Autodesk Inventor part; units mm, degrees
(part 2 of 2)
sketch "ShorterHoneycomb" plane through (90.804, 0, 48.8878) normal (1, 0, 0) x (0, 0, -1)
  line L0 (0, 131) -> (113, 131)
  line L1 (113, 131) -> (113, 0)
  line L2 (113, 0) -> (0, 0)
  line L3 (0, 0) -> (0, 131)
  line L4 (4, 131) -> (109, 131)
  line L5 (109, 131) -> (109, 0)
  line L6 (109, 0) -> (4, 0)
  line L7 (4, 0) -> (4, 131)
  line L8 (15.2583, 115) -> (7.7528, 115)
  line L9 (7.7528, 115) -> (4, 121.5)
  line L10 (4, 121.5) -> (7.7528, 128)
  line L11 (7.7528, 128) -> (15.2583, 128)
  line L12 (15.2583, 128) -> (19.0111, 121.5)
  line L13 (19.0111, 121.5) -> (15.2583, 115)
  line L14 (27.094, 107.5) -> (19.5885, 107.5)
  line L15 (19.5885, 107.5) -> (15.8357, 114)
  line L16 (15.8357, 114) -> (19.5885, 120.5)
  line L17 (19.5885, 120.5) -> (27.094, 120.5)
  line L18 (27.094, 120.5) -> (30.8468, 114)
  line L19 (30.8468, 114) -> (27.094, 107.5)
  line L20 (0, 131) -> (113, 131) projected
  line L21 (19.0111, 121.5) -> (19.5885, 120.5) construction
  line L22 (15.2583, 115) -> (15.8357, 114) construction
  line L23 (15.2583, 100) -> (7.7528, 100)
  line L24 (7.7528, 100) -> (4, 106.5)
  line L25 (4, 106.5) -> (7.7528, 113)
  line L26 (7.7528, 113) -> (15.2583, 113)
  line L27 (15.2583, 113) -> (19.0111, 106.5)
  line L28 (19.0111, 106.5) -> (15.2583, 100)
  line L29 (27.094, 92.5) -> (19.5885, 92.5)
  line L30 (19.5885, 92.5) -> (15.8357, 99)
  line L31 (15.8357, 99) -> (19.5885, 105.5)
  line L32 (19.5885, 105.5) -> (27.094, 105.5)
  line L33 (27.094, 105.5) -> (30.8468, 99)
  line L34 (30.8468, 99) -> (27.094, 92.5)
  line L35 (19.0111, 106.5) -> (19.5885, 105.5) construction
  line L36 (15.2583, 100) -> (15.8357, 99) construction
  line L37 (15.2583, 85) -> (7.7528, 85)
  line L38 (7.7528, 85) -> (4, 91.5)
  line L39 (4, 91.5) -> (7.7528, 98)
  line L40 (7.7528, 98) -> (15.2583, 98)
  line L41 (15.2583, 98) -> (19.0111, 91.5)
  line L42 (19.0111, 91.5) -> (15.2583, 85)
  line L43 (27.094, 77.5) -> (19.5885, 77.5)
  line L44 (19.5885, 77.5) -> (15.8357, 84)
  line L45 (15.8357, 84) -> (19.5885, 90.5)
  line L46 (19.5885, 90.5) -> (27.094, 90.5)
  line L47 (27.094, 90.5) -> (30.8468, 84)
  line L48 (30.8468, 84) -> (27.094, 77.5)
  line L49 (19.0111, 91.5) -> (19.5885, 90.5) construction
  line L50 (15.2583, 85) -> (15.8357, 84) construction
  line L51 (15.2583, 70) -> (7.7528, 70)
  line L52 (7.7528, 70) -> (4, 76.5)
  line L53 (4, 76.5) -> (7.7528, 83)
  line L54 (7.7528, 83) -> (15.2583, 83)
  line L55 (15.2583, 83) -> (19.0111, 76.5)
  line L56 (19.0111, 76.5) -> (15.2583, 70)
  line L57 (27.094, 62.5) -> (19.5885, 62.5)
  line L58 (19.5885, 62.5) -> (15.8357, 69)
  line L59 (15.8357, 69) -> (19.5885, 75.5)
  line L60 (19.5885, 75.5) -> (27.094, 75.5)
  line L61 (27.094, 75.5) -> (30.8468, 69)
  line L62 (30.8468, 69) -> (27.094, 62.5)
  line L63 (19.0111, 76.5) -> (19.5885, 75.5) construction
  line L64 (15.2583, 70) -> (15.8357, 69) construction
  line L65 (15.2583, 55) -> (7.7528, 55)
  line L66 (7.7528, 55) -> (4, 61.5)
  line L67 (4, 61.5) -> (7.7528, 68)
  line L68 (7.7528, 68) -> (15.2583, 68)
  line L69 (15.2583, 68) -> (19.0111, 61.5)
  line L70 (19.0111, 61.5) -> (15.2583, 55)
  line L71 (27.094, 47.5) -> (19.5885, 47.5)
  line L72 (19.5885, 47.5) -> (15.8357, 54)
  line L73 (15.8357, 54) -> (19.5885, 60.5)
  line L74 (19.5885, 60.5) -> (27.094, 60.5)
  line L75 (27.094, 60.5) -> (30.8468, 54)
  line L76 (30.8468, 54) -> (27.094, 47.5)
  line L77 (19.0111, 61.5) -> (19.5885, 60.5) construction
  line L78 (15.2583, 55) -> (15.8357, 54) construction
  line L79 (15.2583, 40) -> (7.7528, 40)
  line L80 (7.7528, 40) -> (4, 46.5)
  line L81 (4, 46.5) -> (7.7528, 53)
  line L82 (7.7528, 53) -> (15.2583, 53)
  line L83 (15.2583, 53) -> (19.0111, 46.5)
  line L84 (19.0111, 46.5) -> (15.2583, 40)
  line L85 (27.094, 32.5) -> (19.5885, 32.5)
  line L86 (19.5885, 32.5) -> (15.8357, 39)
  line L87 (15.8357, 39) -> (19.5885, 45.5)
  line L88 (19.5885, 45.5) -> (27.094, 45.5)
  line L89 (27.094, 45.5) -> (30.8468, 39)
  line L90 (30.8468, 39) -> (27.094, 32.5)
  line L91 (19.0111, 46.5) -> (19.5885, 45.5) construction
  line L92 (15.2583, 40) -> (15.8357, 39) construction
  line L93 (15.2583, 25) -> (7.7528, 25)
  line L94 (7.7528, 25) -> (4, 31.5)
  line L95 (4, 31.5) -> (7.7528, 38)
  line L96 (7.7528, 38) -> (15.2583, 38)
  line L97 (15.2583, 38) -> (19.0111, 31.5)
  line L98 (19.0111, 31.5) -> (15.2583, 25)
  line L99 (27.094, 17.5) -> (19.5885, 17.5)
  line L100 (19.5885, 17.5) -> (15.8357, 24)
  line L101 (15.8357, 24) -> (19.5885, 30.5)
  line L102 (19.5885, 30.5) -> (27.094, 30.5)
  line L103 (27.094, 30.5) -> (30.8468, 24)
  line L104 (30.8468, 24) -> (27.094, 17.5)
  line L105 (19.0111, 31.5) -> (19.5885, 30.5) construction
  line L106 (15.2583, 25) -> (15.8357, 24) construction
  line L107 (15.2583, 10) -> (7.7528, 10)
  line L108 (7.7528, 10) -> (4, 16.5)
  line L109 (4, 16.5) -> (7.7528, 23)
  line L110 (7.7528, 23) -> (15.2583, 23)
  line L111 (15.2583, 23) -> (19.0111, 16.5)
  line L112 (19.0111, 16.5) -> (15.2583, 10)
  line L113 (27.094, 2.5) -> (19.5885, 2.5)
  line L114 (19.5885, 2.5) -> (15.8357, 9)
  line L115 (15.8357, 9) -> (19.5885, 15.5)
  line L116 (19.5885, 15.5) -> (27.094, 15.5)
  line L117 (27.094, 15.5) -> (30.8468, 9)
  line L118 (30.8468, 9) -> (27.094, 2.5)
  line L119 (19.0111, 16.5) -> (19.5885, 15.5) construction
  line L120 (15.2583, 10) -> (15.8357, 9) construction
  line L121 (38.9333, 115) -> (31.4278, 115)
  line L122 (31.4278, 115) -> (27.675, 121.5)
  line L123 (27.675, 121.5) -> (31.4278, 128)
  line L124 (31.4278, 128) -> (38.9333, 128)
  line L125 (38.9333, 128) -> (42.6861, 121.5)
  line L126 (42.6861, 121.5) -> (38.9333, 115)
  line L127 (50.769, 107.5) -> (43.2635, 107.5)
  line L128 (43.2635, 107.5) -> (39.5107, 114)
  line L129 (39.5107, 114) -> (43.2635, 120.5)
  line L130 (43.2635, 120.5) -> (50.769, 120.5)
  line L131 (50.769, 120.5) -> (54.5218, 114)
  line L132 (54.5218, 114) -> (50.769, 107.5)
  line L133 (42.6861, 121.5) -> (43.2635, 120.5) construction
  line L134 (38.9333, 115) -> (39.5107, 114) construction
  line L135 (38.9333, 100) -> (31.4278, 100)
  line L136 (31.4278, 100) -> (27.675, 106.5)
  line L137 (27.675, 106.5) -> (31.4278, 113)
  line L138 (31.4278, 113) -> (38.9333, 113)
  line L139 (38.9333, 113) -> (42.6861, 106.5)
  line L140 (42.6861, 106.5) -> (38.9333, 100)
  line L141 (50.769, 92.5) -> (43.2635, 92.5)
  line L142 (43.2635, 92.5) -> (39.5107, 99)
  line L143 (39.5107, 99) -> (43.2635, 105.5)
  line L144 (43.2635, 105.5) -> (50.769, 105.5)
  line L145 (50.769, 105.5) -> (54.5218, 99)
  line L146 (54.5218, 99) -> (50.769, 92.5)
  line L147 (42.6861, 106.5) -> (43.2635, 105.5) construction
  line L148 (38.9333, 100) -> (39.5107, 99) construction
  line L149 (38.9333, 85) -> (31.4278, 85)
  line L150 (31.4278, 85) -> (27.675, 91.5)
  line L151 (27.675, 91.5) -> (31.4278, 98)
  line L152 (31.4278, 98) -> (38.9333, 98)
  line L153 (38.9333, 98) -> (42.6861, 91.5)
  line L154 (42.6861, 91.5) -> (38.9333, 85)
  line L155 (50.769, 77.5) -> (43.2635, 77.5)
  line L156 (43.2635, 77.5) -> (39.5107, 84)
  line L157 (39.5107, 84) -> (43.2635, 90.5)
  line L158 (43.2635, 90.5) -> (50.769, 90.5)
  line L159 (50.769, 90.5) -> (54.5218, 84)
  line L160 (54.5218, 84) -> (50.769, 77.5)
  line L161 (42.6861, 91.5) -> (43.2635, 90.5) construction
  line L162 (38.9333, 85) -> (39.5107, 84) construction
  line L163 (38.9333, 70) -> (31.4278, 70)
  line L164 (31.4278, 70) -> (27.675, 76.5)
  line L165 (27.675, 76.5) -> (31.4278, 83)
  line L166 (31.4278, 83) -> (38.9333, 83)
  line L167 (38.9333, 83) -> (42.6861, 76.5)
  line L168 (42.6861, 76.5) -> (38.9333, 70)
  line L169 (50.769, 62.5) -> (43.2635, 62.5)
  line L170 (43.2635, 62.5) -> (39.5107, 69)
  line L171 (39.5107, 69) -> (43.2635, 75.5)
  line L172 (43.2635, 75.5) -> (50.769, 75.5)
  line L173 (50.769, 75.5) -> (54.5218, 69)
  line L174 (54.5218, 69) -> (50.769, 62.5)
  line L175 (42.6861, 76.5) -> (43.2635, 75.5) construction
  line L176 (38.9333, 70) -> (39.5107, 69) construction
  line L177 (38.9333, 55) -> (31.4278, 55)
  line L178 (31.4278, 55) -> (27.675, 61.5)
  line L179 (27.675, 61.5) -> (31.4278, 68)
  line L180 (31.4278, 68) -> (38.9333, 68)
  line L181 (38.9333, 68) -> (42.6861, 61.5)
  line L182 (42.6861, 61.5) -> (38.9333, 55)
  line L183 (50.769, 47.5) -> (43.2635, 47.5)
  line L184 (43.2635, 47.5) -> (39.5107, 54)
  line L185 (39.5107, 54) -> (43.2635, 60.5)
  line L186 (43.2635, 60.5) -> (50.769, 60.5)
  line L187 (50.769, 60.5) -> (54.5218, 54)
  line L188 (54.5218, 54) -> (50.769, 47.5)
  line L189 (42.6861, 61.5) -> (43.2635, 60.5) construction
  line L190 (38.9333, 55) -> (39.5107, 54) construction
  line L191 (38.9333, 40) -> (31.4278, 40)
  line L192 (31.4278, 40) -> (27.675, 46.5)
  line L193 (27.675, 46.5) -> (31.4278, 53)
  line L194 (31.4278, 53) -> (38.9333, 53)
  line L195 (38.9333, 53) -> (42.6861, 46.5)
  line L196 (42.6861, 46.5) -> (38.9333, 40)
  line L197 (50.769, 32.5) -> (43.2635, 32.5)
  line L198 (43.2635, 32.5) -> (39.5107, 39)
  line L199 (39.5107, 39) -> (43.2635, 45.5)
  line L200 (43.2635, 45.5) -> (50.769, 45.5)
  line L201 (50.769, 45.5) -> (54.5218, 39)
  line L202 (54.5218, 39) -> (50.769, 32.5)
  line L203 (42.6861, 46.5) -> (43.2635, 45.5) construction
  line L204 (38.9333, 40) -> (39.5107, 39) construction
  line L205 (38.9333, 25) -> (31.4278, 25)
  line L206 (31.4278, 25) -> (27.675, 31.5)
  line L207 (27.675, 31.5) -> (31.4278, 38)
  line L208 (31.4278, 38) -> (38.9333, 38)
  line L209 (38.9333, 38) -> (42.6861, 31.5)
  line L210 (42.6861, 31.5) -> (38.9333, 25)
  line L211 (50.769, 17.5) -> (43.2635, 17.5)
  line L212 (43.2635, 17.5) -> (39.5107, 24)
  line L213 (39.5107, 24) -> (43.2635, 30.5)
  line L214 (43.2635, 30.5) -> (50.769, 30.5)
  line L215 (50.769, 30.5) -> (54.5218, 24)
  line L216 (54.5218, 24) -> (50.769, 17.5)
  line L217 (42.6861, 31.5) -> (43.2635, 30.5) construction
  line L218 (38.9333, 25) -> (39.5107, 24) construction
  line L219 (38.9333, 10) -> (31.4278, 10)
  line L220 (31.4278, 10) -> (27.675, 16.5)
  line L221 (27.675, 16.5) -> (31.4278, 23)
  line L222 (31.4278, 23) -> (38.9333, 23)
  line L223 (38.9333, 23) -> (42.6861, 16.5)
  line L224 (42.6861, 16.5) -> (38.9333, 10)
  line L225 (50.769, 2.5) -> (43.2635, 2.5)
  line L226 (43.2635, 2.5) -> (39.5107, 9)
  line L227 (39.5107, 9) -> (43.2635, 15.5)
  line L228 (43.2635, 15.5) -> (50.769, 15.5)
  line L229 (50.769, 15.5) -> (54.5218, 9)
  line L230 (54.5218, 9) -> (50.769, 2.5)
  line L231 (42.6861, 16.5) -> (43.2635, 15.5) construction
  line L232 (38.9333, 10) -> (39.5107, 9) construction
  line L233 (62.6083, 115) -> (55.1028, 115)
  line L234 (55.1028, 115) -> (51.35, 121.5)
  line L235 (51.35, 121.5) -> (55.1028, 128)
  line L236 (55.1028, 128) -> (62.6083, 128)
  line L237 (62.6083, 128) -> (66.3611, 121.5)
  line L238 (66.3611, 121.5) -> (62.6083, 115)
  line L239 (74.444, 107.5) -> (66.9385, 107.5)
  line L240 (66.9385, 107.5) -> (63.1857, 114)
  line L241 (63.1857, 114) -> (66.9385, 120.5)
  line L242 (66.9385, 120.5) -> (74.444, 120.5)
  line L243 (74.444, 120.5) -> (78.1968, 114)
  line L244 (78.1968, 114) -> (74.444, 107.5)
  line L245 (66.3611, 121.5) -> (66.9385, 120.5) construction
  line L246 (62.6083, 115) -> (63.1857, 114) construction
  line L247 (62.6083, 100) -> (55.1028, 100)
  line L248 (55.1028, 100) -> (51.35, 106.5)
  line L249 (51.35, 106.5) -> (55.1028, 113)
  line L250 (55.1028, 113) -> (62.6083, 113)
  line L251 (62.6083, 113) -> (66.3611, 106.5)
  line L252 (66.3611, 106.5) -> (62.6083, 100)
  line L253 (74.444, 92.5) -> (66.9385, 92.5)
  line L254 (66.9385, 92.5) -> (63.1857, 99)
  line L255 (63.1857, 99) -> (66.9385, 105.5)
  line L256 (66.9385, 105.5) -> (74.444, 105.5)
  line L257 (74.444, 105.5) -> (78.1968, 99)
  line L258 (78.1968, 99) -> (74.444, 92.5)
  line L259 (66.3611, 106.5) -> (66.9385, 105.5) construction
  line L260 (62.6083, 100) -> (63.1857, 99) construction
  line L261 (62.6083, 85) -> (55.1028, 85)
  line L262 (55.1028, 85) -> (51.35, 91.5)
  line L263 (51.35, 91.5) -> (55.1028, 98)
  line L264 (55.1028, 98) -> (62.6083, 98)
  line L265 (62.6083, 98) -> (66.3611, 91.5)
  line L266 (66.3611, 91.5) -> (62.6083, 85)
  line L267 (74.444, 77.5) -> (66.9385, 77.5)
  line L268 (66.9385, 77.5) -> (63.1857, 84)
  line L269 (63.1857, 84) -> (66.9385, 90.5)
  line L270 (66.9385, 90.5) -> (74.444, 90.5)
  line L271 (74.444, 90.5) -> (78.1968, 84)
  line L272 (78.1968, 84) -> (74.444, 77.5)
  line L273 (66.3611, 91.5) -> (66.9385, 90.5) construction
  line L274 (62.6083, 85) -> (63.1857, 84) construction
  line L275 (62.6083, 70) -> (55.1028, 70)
  line L276 (55.1028, 70) -> (51.35, 76.5)
  line L277 (51.35, 76.5) -> (55.1028, 83)
  line L278 (55.1028, 83) -> (62.6083, 83)
  line L279 (62.6083, 83) -> (66.3611, 76.5)
  line L280 (66.3611, 76.5) -> (62.6083, 70)
  line L281 (74.444, 62.5) -> (66.9385, 62.5)
  line L282 (66.9385, 62.5) -> (63.1857, 69)
  line L283 (63.1857, 69) -> (66.9385, 75.5)
  line L284 (66.9385, 75.5) -> (74.444, 75.5)
  line L285 (74.444, 75.5) -> (78.1968, 69)
  line L286 (78.1968, 69) -> (74.444, 62.5)
  line L287 (66.3611, 76.5) -> (66.9385, 75.5) construction
  line L288 (62.6083, 70) -> (63.1857, 69) construction
  line L289 (62.6083, 55) -> (55.1028, 55)
  line L290 (55.1028, 55) -> (51.35, 61.5)
  line L291 (51.35, 61.5) -> (55.1028, 68)
  line L292 (55.1028, 68) -> (62.6083, 68)
  line L293 (62.6083, 68) -> (66.3611, 61.5)
  line L294 (66.3611, 61.5) -> (62.6083, 55)
  line L295 (74.444, 47.5) -> (66.9385, 47.5)
  line L296 (66.9385, 47.5) -> (63.1857, 54)
  line L297 (63.1857, 54) -> (66.9385, 60.5)
  line L298 (66.9385, 60.5) -> (74.444, 60.5)
  line L299 (74.444, 60.5) -> (78.1968, 54)
  line L300 (78.1968, 54) -> (74.444, 47.5)
  line L301 (66.3611, 61.5) -> (66.9385, 60.5) construction
  line L302 (62.6083, 55) -> (63.1857, 54) construction
  line L303 (62.6083, 40) -> (55.1028, 40)
  line L304 (55.1028, 40) -> (51.35, 46.5)
  line L305 (51.35, 46.5) -> (55.1028, 53)
  line L306 (55.1028, 53) -> (62.6083, 53)
  line L307 (62.6083, 53) -> (66.3611, 46.5)
  line L308 (66.3611, 46.5) -> (62.6083, 40)
  line L309 (74.444, 32.5) -> (66.9385, 32.5)
  line L310 (66.9385, 32.5) -> (63.1857, 39)
  line L311 (63.1857, 39) -> (66.9385, 45.5)
  line L312 (66.9385, 45.5) -> (74.444, 45.5)
  line L313 (74.444, 45.5) -> (78.1968, 39)
  line L314 (78.1968, 39) -> (74.444, 32.5)
  line L315 (66.3611, 46.5) -> (66.9385, 45.5) construction
  line L316 (62.6083, 40) -> (63.1857, 39) construction
  line L317 (62.6083, 25) -> (55.1028, 25)
  line L318 (55.1028, 25) -> (51.35, 31.5)
  line L319 (51.35, 31.5) -> (55.1028, 38)
  line L320 (55.1028, 38) -> (62.6083, 38)
  line L321 (62.6083, 38) -> (66.3611, 31.5)
  line L322 (66.3611, 31.5) -> (62.6083, 25)
  line L323 (74.444, 17.5) -> (66.9385, 17.5)
  line L324 (66.9385, 17.5) -> (63.1857, 24)
  line L325 (63.1857, 24) -> (66.9385, 30.5)
  line L326 (66.9385, 30.5) -> (74.444, 30.5)
  line L327 (74.444, 30.5) -> (78.1968, 24)
  line L328 (78.1968, 24) -> (74.444, 17.5)
  line L329 (66.3611, 31.5) -> (66.9385, 30.5) construction
  line L330 (62.6083, 25) -> (63.1857, 24) construction
  line L331 (62.6083, 10) -> (55.1028, 10)
  line L332 (55.1028, 10) -> (51.35, 16.5)
  line L333 (51.35, 16.5) -> (55.1028, 23)
  line L334 (55.1028, 23) -> (62.6083, 23)
  line L335 (62.6083, 23) -> (66.3611, 16.5)
  line L336 (66.3611, 16.5) -> (62.6083, 10)
  line L337 (74.444, 2.5) -> (66.9385, 2.5)
  line L338 (66.9385, 2.5) -> (63.1857, 9)
  line L339 (63.1857, 9) -> (66.9385, 15.5)
  line L340 (66.9385, 15.5) -> (74.444, 15.5)
  line L341 (74.444, 15.5) -> (78.1968, 9)
  line L342 (78.1968, 9) -> (74.444, 2.5)
  line L343 (66.3611, 16.5) -> (66.9385, 15.5) construction
  line L344 (62.6083, 10) -> (63.1857, 9) construction
  line L345 (86.2833, 115) -> (78.7778, 115)
  line L346 (78.7778, 115) -> (75.025, 121.5)
  line L347 (75.025, 121.5) -> (78.7778, 128)
  line L348 (78.7778, 128) -> (86.2833, 128)
  line L349 (86.2833, 128) -> (90.0361, 121.5)
  line L350 (90.0361, 121.5) -> (86.2833, 115)
  line L351 (98.119, 107.5) -> (90.6135, 107.5)
  line L352 (90.6135, 107.5) -> (86.8607, 114)
  line L353 (86.8607, 114) -> (90.6135, 120.5)
  line L354 (90.6135, 120.5) -> (98.119, 120.5)
  line L355 (98.119, 120.5) -> (101.8718, 114)
  line L356 (101.8718, 114) -> (98.119, 107.5)
  line L357 (90.0361, 121.5) -> (90.6135, 120.5) construction
  line L358 (86.2833, 115) -> (86.8607, 114) construction
  line L359 (86.2833, 100) -> (78.7778, 100)
  line L360 (78.7778, 100) -> (75.025, 106.5)
  line L361 (75.025, 106.5) -> (78.7778, 113)
  line L362 (78.7778, 113) -> (86.2833, 113)
  line L363 (86.2833, 113) -> (90.0361, 106.5)
  line L364 (90.0361, 106.5) -> (86.2833, 100)
  line L365 (98.119, 92.5) -> (90.6135, 92.5)
  line L366 (90.6135, 92.5) -> (86.8607, 99)
  line L367 (86.8607, 99) -> (90.6135, 105.5)
  line L368 (90.6135, 105.5) -> (98.119, 105.5)
  line L369 (98.119, 105.5) -> (101.8718, 99)
  line L370 (101.8718, 99) -> (98.119, 92.5)
  line L371 (90.0361, 106.5) -> (90.6135, 105.5) construction
  line L372 (86.2833, 100) -> (86.8607, 99) construction
  line L373 (86.2833, 85) -> (78.7778, 85)
  line L374 (78.7778, 85) -> (75.025, 91.5)
  line L375 (75.025, 91.5) -> (78.7778, 98)
  line L376 (78.7778, 98) -> (86.2833, 98)
  line L377 (86.2833, 98) -> (90.0361, 91.5)
  line L378 (90.0361, 91.5) -> (86.2833, 85)
  line L379 (98.119, 77.5) -> (90.6135, 77.5)
  line L380 (90.6135, 77.5) -> (86.8607, 84)
  line L381 (86.8607, 84) -> (90.6135, 90.5)
  line L382 (90.6135, 90.5) -> (98.119, 90.5)
  line L383 (98.119, 90.5) -> (101.8718, 84)
  line L384 (101.8718, 84) -> (98.119, 77.5)
  line L385 (90.0361, 91.5) -> (90.6135, 90.5) construction
  line L386 (86.2833, 85) -> (86.8607, 84) construction
  line L387 (86.2833, 70) -> (78.7778, 70)
  line L388 (78.7778, 70) -> (75.025, 76.5)
  line L389 (75.025, 76.5) -> (78.7778, 83)
  line L390 (78.7778, 83) -> (86.2833, 83)
  line L391 (86.2833, 83) -> (90.0361, 76.5)
  line L392 (90.0361, 76.5) -> (86.2833, 70)
  line L393 (98.119, 62.5) -> (90.6135, 62.5)
  line L394 (90.6135, 62.5) -> (86.8607, 69)
  line L395 (86.8607, 69) -> (90.6135, 75.5)
  line L396 (90.6135, 75.5) -> (98.119, 75.5)
  line L397 (98.119, 75.5) -> (101.8718, 69)
  line L398 (101.8718, 69) -> (98.119, 62.5)
  line L399 (90.0361, 76.5) -> (90.6135, 75.5) construction
  line L400 (86.2833, 70) -> (86.8607, 69) construction
  line L401 (86.2833, 55) -> (78.7778, 55)
  line L402 (78.7778, 55) -> (75.025, 61.5)
  line L403 (75.025, 61.5) -> (78.7778, 68)
  line L404 (78.7778, 68) -> (86.2833, 68)
  line L405 (86.2833, 68) -> (90.0361, 61.5)
  line L406 (90.0361, 61.5) -> (86.2833, 55)
  line L407 (98.119, 47.5) -> (90.6135, 47.5)
  line L408 (90.6135, 47.5) -> (86.8607, 54)
  line L409 (86.8607, 54) -> (90.6135, 60.5)
  line L410 (90.6135, 60.5) -> (98.119, 60.5)
  line L411 (98.119, 60.5) -> (101.8718, 54)
  line L412 (101.8718, 54) -> (98.119, 47.5)
  line L413 (90.0361, 61.5) -> (90.6135, 60.5) construction
  line L414 (86.2833, 55) -> (86.8607, 54) construction
  line L415 (86.2833, 40) -> (78.7778, 40)
  line L416 (78.7778, 40) -> (75.025, 46.5)
  line L417 (75.025, 46.5) -> (78.7778, 53)
  line L418 (78.7778, 53) -> (86.2833, 53)
  line L419 (86.2833, 53) -> (90.0361, 46.5)
  line L420 (90.0361, 46.5) -> (86.2833, 40)
  line L421 (98.119, 32.5) -> (90.6135, 32.5)
  line L422 (90.6135, 32.5) -> (86.8607, 39)
  line L423 (86.8607, 39) -> (90.6135, 45.5)
  line L424 (90.6135, 45.5) -> (98.119, 45.5)
  line L425 (98.119, 45.5) -> (101.8718, 39)
  line L426 (101.8718, 39) -> (98.119, 32.5)
  line L427 (90.0361, 46.5) -> (90.6135, 45.5) construction
  line L428 (86.2833, 40) -> (86.8607, 39) construction
  line L429 (86.2833, 25) -> (78.7778, 25)
  line L430 (78.7778, 25) -> (75.025, 31.5)
  line L431 (75.025, 31.5) -> (78.7778, 38)
  line L432 (78.7778, 38) -> (86.2833, 38)
  line L433 (86.2833, 38) -> (90.0361, 31.5)
  line L434 (90.0361, 31.5) -> (86.2833, 25)
  line L435 (98.119, 17.5) -> (90.6135, 17.5)
  line L436 (90.6135, 17.5) -> (86.8607, 24)
  line L437 (86.8607, 24) -> (90.6135, 30.5)
  line L438 (90.6135, 30.5) -> (98.119, 30.5)
  line L439 (98.119, 30.5) -> (101.8718, 24)
  line L440 (101.8718, 24) -> (98.119, 17.5)
  line L441 (90.0361, 31.5) -> (90.6135, 30.5) construction
  line L442 (86.2833, 25) -> (86.8607, 24) construction
  line L443 (86.2833, 10) -> (78.7778, 10)
  line L444 (78.7778, 10) -> (75.025, 16.5)
  line L445 (75.025, 16.5) -> (78.7778, 23)
  line L446 (78.7778, 23) -> (86.2833, 23)
  line L447 (86.2833, 23) -> (90.0361, 16.5)
  line L448 (90.0361, 16.5) -> (86.2833, 10)
  line L449 (98.119, 2.5) -> (90.6135, 2.5)
  line L450 (90.6135, 2.5) -> (86.8607, 9)
  line L451 (86.8607, 9) -> (90.6135, 15.5)
  line L452 (90.6135, 15.5) -> (98.119, 15.5)
  line L453 (98.119, 15.5) -> (101.8718, 9)
  line L454 (101.8718, 9) -> (98.119, 2.5)
  line L455 (90.0361, 16.5) -> (90.6135, 15.5) construction
  line L456 (86.2833, 10) -> (86.8607, 9) construction
  line L457 (109.9583, 115) -> (102.4528, 115)
  line L458 (102.4528, 115) -> (98.7, 121.5)
  line L459 (102.4528, 128) -> (109.9583, 128)
  line L460 (109.9583, 128) -> (113.7111, 121.5)
  line L461 (113.7111, 121.5) -> (109.9583, 115)
  line L462 (98.7, 121.5) -> (102.4528, 128)
  line L463 (109.9583, 100) -> (102.4528, 100)
  line L464 (102.4528, 100) -> (98.7, 106.5)
  line L465 (102.4528, 113) -> (109.9583, 113)
  line L466 (109.9583, 113) -> (113.7111, 106.5)
  line L467 (113.7111, 106.5) -> (109.9583, 100)
  line L468 (98.7, 106.5) -> (102.4528, 113)
  line L469 (109.9583, 85) -> (102.4528, 85)
  line L470 (102.4528, 85) -> (98.7, 91.5)
  line L471 (102.4528, 98) -> (109.9583, 98)
  line L472 (109.9583, 98) -> (113.7111, 91.5)
  line L473 (113.7111, 91.5) -> (109.9583, 85)
  line L474 (98.7, 91.5) -> (102.4528, 98)
  line L475 (109.9583, 70) -> (102.4528, 70)
  line L476 (102.4528, 70) -> (98.7, 76.5)
  line L477 (102.4528, 83) -> (109.9583, 83)
  line L478 (109.9583, 83) -> (113.7111, 76.5)
  line L479 (113.7111, 76.5) -> (109.9583, 70)
  line L480 (98.7, 76.5) -> (102.4528, 83)
  line L481 (109.9583, 55) -> (102.4528, 55)
  line L482 (102.4528, 55) -> (98.7, 61.5)
  line L483 (102.4528, 68) -> (109.9583, 68)
  line L484 (109.9583, 68) -> (113.7111, 61.5)
  line L485 (113.7111, 61.5) -> (109.9583, 55)
  line L486 (98.7, 61.5) -> (102.4528, 68)
  line L487 (109.9583, 40) -> (102.4528, 40)
  line L488 (102.4528, 40) -> (98.7, 46.5)
  line L489 (102.4528, 53) -> (109.9583, 53)
  line L490 (109.9583, 53) -> (113.7111, 46.5)
  line L491 (113.7111, 46.5) -> (109.9583, 40)
  line L492 (98.7, 46.5) -> (102.4528, 53)
  line L493 (109.9583, 25) -> (102.4528, 25)
  line L494 (102.4528, 25) -> (98.7, 31.5)
  line L495 (102.4528, 38) -> (109.9583, 38)
  line L496 (109.9583, 38) -> (113.7111, 31.5)
  line L497 (113.7111, 31.5) -> (109.9583, 25)
  line L498 (98.7, 31.5) -> (102.4528, 38)
  line L499 (109.9583, 10) -> (102.4528, 10)
  line L500 (102.4528, 10) -> (98.7, 16.5)
  line L501 (102.4528, 23) -> (109.9583, 23)
  line L502 (109.9583, 23) -> (113.7111, 16.5)
  line L503 (113.7111, 16.5) -> (109.9583, 10)
  line L504 (98.7, 16.5) -> (102.4528, 23)
  point P0 (48.8878, 0)
  point P1 (11.5056, 121.5)
  point P2 (23.3412, 114)
  point P3 (11.5056, 106.5)
  point P4 (23.3412, 99)
  point P5 (11.5056, 91.5)
  point P6 (23.3412, 84)
  point P7 (11.5056, 76.5)
  point P8 (23.3412, 69)
  point P9 (11.5056, 61.5)
  point P10 (23.3412, 54)
  point P11 (11.5056, 46.5)
  point P12 (23.3412, 39)
  point P13 (11.5056, 31.5)
  point P14 (23.3412, 24)
  point P15 (11.5056, 16.5)
  point P16 (23.3412, 9)
  point P17 (35.1806, 121.5)
  point P18 (47.0162, 114)
  point P19 (35.1806, 106.5)
  point P20 (47.0162, 99)
  point P21 (35.1806, 91.5)
  point P22 (47.0162, 84)
  point P23 (35.1806, 76.5)
  point P24 (47.0162, 69)
  point P25 (35.1806, 61.5)
  point P26 (47.0162, 54)
  point P27 (35.1806, 46.5)
  point P28 (47.0162, 39)
  point P29 (35.1806, 31.5)
  point P30 (47.0162, 24)
  point P31 (35.1806, 16.5)
  point P32 (47.0162, 9)
  point P33 (58.8556, 121.5)
  point P34 (70.6912, 114)
  point P35 (58.8556, 106.5)
  point P36 (70.6912, 99)
  point P37 (58.8556, 91.5)
  point P38 (70.6912, 84)
  point P39 (58.8556, 76.5)
  point P40 (70.6912, 69)
  point P41 (58.8556, 61.5)
  point P42 (70.6912, 54)
  point P43 (58.8556, 46.5)
  point P44 (70.6912, 39)
  point P45 (58.8556, 31.5)
  point P46 (70.6912, 24)
  point P47 (58.8556, 16.5)
  point P48 (70.6912, 9)
  point P49 (82.5306, 121.5)
  point P50 (94.3662, 114)
  point P51 (82.5306, 106.5)
  point P52 (94.3662, 99)
  point P53 (82.5306, 91.5)
  point P54 (94.3662, 84)
  point P55 (82.5306, 76.5)
  point P56 (94.3662, 69)
  point P57 (82.5306, 61.5)
  point P58 (94.3662, 54)
  point P59 (82.5306, 46.5)
  point P60 (94.3662, 39)
  point P61 (82.5306, 31.5)
  point P62 (94.3662, 24)
  point P63 (82.5306, 16.5)
  point P64 (94.3662, 9)
  point P65 (106.2056, 121.5)
  dimension "d32" = 13
  dimension "d33" = 1
  dimension "d35" = 3
  dimension "d36" = 0
  dimension "d39" = 15
  dimension "d42" = 23.675
  dimension "d56" = 1
  dimension "d57" = 2
  dimension "d58" = 1
  dimension "d59" = 1.0031
  dimension "d62" = 23.675
  dimension "d137" = 1
  dimension "d138" = 1.0031
  dimension "d139" = 1.0031
  dimension "d140" = 2
  constraints: 1008 end point, 7 parallel, 4 horizontal, 2 collinear, 2 perpendicular, 1 vertical, 991 other
  measures "d32" distance between parallel lines of L8 L11
  measures "d33" distance between parallel lines of L16 L13
  measures "d35" distance between parallel lines of L4 L11
  measures "d36" distance from line of L7 L9.end
  measures "d39" distance of L14.end L29.end
  measures "d42" distance of L14.end L127.end
  measures "d56" distance between parallel lines of L381 L378
  measures "d57" distance between parallel lines of L376 L359
  measures "d58" distance between parallel lines of L366 L377
  measures "d59" distance between parallel lines of L258 L375
  measures "d62" distance of point (82.531, 121.5) point (106.206, 121.5)
  measures "d137" distance between parallel lines of L27 L15
  measures "d138" distance between parallel lines of L137 L19
  measures "d139" distance between parallel lines of L18 L122
  measures "d140" distance between parallel lines of L26 L8
extrude "HoneycombShortSide" cut sketch "ShorterHoneycomb" against normal blind 200 contours L10 L11 L12 L13 L8 L9 | L25 L26 L27 L28 L23 L24 | L39 L40 L41 L42 L37 L38 | L53 L54 L55 L56 L51 L52 | L67 L68 L69 L70 L65 L66 | L81 L82 L83 L84 L79 L80 | L95 L96 L97 L98 L93 L94 | L109 L110 L111 L112 L107 L108 | L14 L15 L16 L17 L18 L19 | L29 L30 L31 L32 L33 L34 | L43 L44 L45 L46 L47 L48 | L57 L58 L59 L60 L61 L62 | L71 L72 L73 L74 L75 L76 | L85 L86 L87 L88 L89 L90 | L99 L100 L101 L102 L103 L104 | L113 L114 L115 L116 L117 L118 | L121 L122 L123 L124 L125 L126 | L127 L128 L129 L130 L131 L132 | L135 L136 L137 L138 L139 L140 | L141 L142 L143 L144 L145 L146 | L149 L150 L151 L152 L153 L154 | L155 L156 L157 L158 L159 L160 | L163 L164 L165 L166 L167 L168 | L169 L170 L171 L172 L173 L174 | L177 L178 L179 L180 L181 L182 | L183 L184 L185 L186 L187 L188 | L191 L192 L193 L194 L195 L196 | L197 L198 L199 L200 L201 L202 | L205 L206 L207 L208 L209 L210 | L211 L212 L213 L214 L215 L216 | L219 L220 L221 L222 L223 L224 | L225 L226 L227 L228 L229 L230 | L233 L234 L235 L236 L237 L238 | L239 L240 L241 L242 L243 L244 | L247 L248 L249 L250 L251 L252 | L253 L254 L255 L256 L257 L258 | L261 L262 L263 L264 L265 L266 | L267 L268 L269 L270 L271 L272 | L275 L276 L277 L278 L279 L280 | L281 L282 L283 L284 L285 L286 | L289 L290 L291 L292 L293 L294 | L295 L296 L297 L298 L299 L300 | L303 L304 L305 L306 L307 L308 | L309 L310 L311 L312 L313 L314 | L317 L318 L319 L320 L321 L322 | L323 L324 L325 L326 L327 L328 | L331 L332 L333 L334 L335 L336 | L337 L338 L339 L340 L341 L342 | L345 L346 L347 L348 L349 L350 | L351 L352 L353 L354 L355 L356 | L359 L360 L361 L362 L363 L364 | L365 L366 L367 L368 L369 L370 | L373 L374 L375 L376 L377 L378 | L379 L380 L381 L382 L383 L384 | L387 L388 L389 L390 L391 L392 | L393 L394 L395 L396 L397 L398 | L401 L402 L403 L404 L405 L406 | L407 L408 L409 L410 L411 L412 | L415 L416 L417 L418 L419 L420 | L421 L422 L423 L424 L425 L426 | L429 L430 L431 L432 L433 L434 | L435 L436 L437 L438 L439 L440 | L443 L444 L445 L446 L447 L448 | L449 L450 L451 L452 L453 L454
extrude "SidePanels" add sketch "BasicBox" along normal blind 131 contours L0 L42 L22 L18 L43 L3 | L43 L18 L40 L3 | L0 L1 L2 L44 L27 L25 L16 L24 L23 L17 L22 L42 | L40 L18 L26 L19 L27 L44 L2 L3
sketch "DroneAttachmentSide1" plane through (-92.196, 0, 48.8878) normal (0, 0, 1) x (1, 0, 0)
  circle A0 centre (51.5, 138) radius 3.5
  circle A1 centre (131.5, 138) radius 3.5
  line L0 (51.5, 138) -> (131.5, 138) construction
  line L1 (0, 131) -> (183, 131) projected
  line L2 (51.5, 138) -> (51.5, 131) construction
  line L3 (179, 131) -> (4, 131) projected
  line L4 (131.5, 138) -> (131.5, 131) construction
  line L5 (0, 131) -> (51.5, 138)
  line L6 (131.5, 138) -> (183, 131)
  arc A2 (61.5, 138) -> (41.5911, 136.6532) centre (51.5, 138) ccw
  line L7 (61.5, 138) -> (67.3737, 131)
  line L8 (61.5, 138) -> (70.6379, 138) construction
  line L9 (0, 131) -> (67.3737, 131)
  arc A3 (141.4089, 136.6532) -> (121.5, 138) centre (131.5, 138) ccw
  line L10 (121.5, 138) -> (113.1577, 131)
  line L11 (121.5, 138) -> (130.7015, 138) construction
  line L12 (113.1577, 131) -> (183, 131)
  line L13 (183, 131) -> (0, 131) projected
  line L14 (0, 0) -> (183, 0) projected
  point P0 (92.196, 0)
  dimension "d72" = 7
  dimension "d73" = 80
  dimension "d74" = 7
  dimension "d75" = 10
  dimension "d76" = 50
  dimension "d77" = 140
  dimension "d133" = 138
  constraints: 22 end point, 6 point on line, 4 centre point, 4 collinear, 4 point on circle, 2 coincident, 2 equal length, 2 equal radius, 2 horizontal, 2 perpendicular, 1 parallel
  measures "d72" diameter of A0
  measures "d73" distance of L0.start L0.end
  measures "d74" distance of L2.end L0.start
  measures "d75" radius of A2
  measures "d76" angle of L7 L8
  measures "d77" angle of L10 L11
  measures "d133" distance from line of L14 A2.centre
extrude "DroneAttachment1" add sketch "DroneAttachmentSide1" against normal blind 4
sketch "Sketch5" plane through (90.804, 0, -64.1122) normal (0, 0, -1) x (-1, 0, 0)
  circle A0 centre (51.5, 138) radius 3.5 projected
  circle A1 centre (51.5, 138) radius 3.5
  circle A2 centre (131.5, 138) radius 3.5 projected
  circle A3 centre (131.5, 138) radius 3.5
  line L0 (69.8423, 131) -> (0, 131)
  line L1 (0, 131) -> (41.5911, 136.6532)
  line L2 (0, 131) -> (41.5911, 136.6532) projected
  line L3 (69.8423, 131) -> (61.5, 138)
  line L4 (69.8423, 131) -> (61.5, 138) projected
  arc A4 (61.5, 138) -> (41.5911, 136.6532) centre (51.5, 138) ccw
  line L5 (121.5, 138) -> (115.6263, 131)
  line L6 (121.5, 138) -> (115.6263, 131) projected
  line L7 (115.6263, 131) -> (183, 131)
  line L8 (183, 131) -> (141.4089, 136.6532)
  line L9 (183, 131) -> (141.4089, 136.6532) projected
  arc A5 (141.4089, 136.6532) -> (121.5, 138) centre (131.5, 138) ccw
  point P0 (90.804, 0)
  constraints: 12 end point, 4 centre point, 4 coincident, 4 collinear, 4 point on circle, 2 horizontal
extrude "Droneattachment2" add sketch "Sketch5" against normal blind 4
sketch "PowerButton" plane through (90.804, 0, 48.8878) normal (1, 0, 0) x (0, 0, -1)
  line L0 (0, 131) -> (113, 131)
  line L1 (113, 131) -> (113, 0)
  line L2 (113, 0) -> (0, 0)
  line L3 (0, 0) -> (0, 131)
  line L4 (4, 131) -> (109, 131)
  line L5 (109, 131) -> (109, 0)
  line L6 (109, 0) -> (4, 0)
  line L7 (4, 0) -> (4, 131)
  circle A0 centre (24, 61) radius 9.5
  point P0 (48.8878, 0)
  dimension "d82" = 19
  dimension "d83" = 20
  dimension "d84" = 70
  constraints: 16 end point, 4 parallel, 2 horizontal, 2 perpendicular, 1 centre point
  measures "d82" diameter of A0
  measures "d83" distance from line of L7 A0.centre
  measures "d84" distance from line of L0 A0.centre
extrude "PowerButtonSupport" add sketch "PowerButton" against normal blind 7 contours A0
hole "PowerButtonHole" at (90.804, 61, 24.8878) direction (-1, 0, 0) diameter 15.7 depth 20 tip angle 118
extrude "LensplateMount" add sketch "BasicBox" along normal blind 15 contours L3 L58 L0 | L58 L59 L60 L61 L62 L0 | L3 L39 L38 L0 L62 L61 L60 L59 | L40 L18 L26 L19 L27 L44 L2 L3 | L3 L64 L69 L68 L67 L2 L41 L40 | L36 L37 L1 L55 L54 L53 L52 L0 | L65 L2 L67 L68 L69 L64 | L3 L2 L65 | L45 L7 L6 L44 L27 L19 L26 L18 | L52 L53 L54 L55 L56 L0 | L56 L1 L0 | L2 L47 L46 L51 L50 L1 L35 L34 | L2 L49 L50 L51 L46 L47 | L49 L2 L1 | A1 | A3
extrude "LensplateaAttachment" add sketch "BasicBox" along normal blind 20 contours L3 L58 L0 | L3 L39 L38 L0 L62 L61 L60 L59 | L40 L18 L26 L19 L27 L44 L2 L3 | L3 L64 L69 L68 L67 L2 L41 L40 | L36 L37 L1 L55 L54 L53 L52 L0 | L3 L2 L65 | L45 L7 L6 L44 L27 L19 L26 L18 | L56 L1 L0 | L2 L47 L46 L51 L50 L1 L35 L34 | L49 L2 L1
sketch "stuffplate_Mount" plane through (-92.196, 0, 48.8878) normal (0, 0, 1) x (1, 0, 0)
  line L0 (0, 131) -> (183, 131)
  line L1 (183, 131) -> (183, 0)
  line L2 (183, 0) -> (0, 0)
  line L3 (0, 0) -> (0, 131)
  line L4 (0, 106) -> (183, 106)
  line L5 (0, 98) -> (183, 98)
  circle A0 centre (75, 102) radius 3
  circle A1 centre (135, 102) radius 3
  line L6 (75, 102) -> (135, 102) construction
  line L7 (148.594, 77.5) -> (141.0885, 77.5) projected
  line L8 (113.0583, 85) -> (105.5528, 85) projected
  line L9 (135, 102) -> (183, 102) construction
  line L10 (183, 84) -> (183, 77.5) projected
  line L11 (75, 102) -> (0, 102) construction
  line L12 (0, 76.5) -> (0, 83) projected
  line L13 (75, 102) -> (75, 98) construction
  line L14 (75, 102) -> (75, 106) construction
  line L15 (135, 102) -> (135, 106) construction
  line L16 (135, 102) -> (135, 98) construction
  point P0 (92.196, 0)
  dimension "d111" = 8
  dimension "d112" = 6
  dimension "d116" = 48
  dimension "d117" = 60
  dimension "d118" = 75
  dimension "d119" = 25
  constraints: 26 end point, 12 point on line, 5 parallel, 5 perpendicular, 2 centre point, 2 equal length, 2 horizontal, 1 equal radius
  measures "d111" distance between parallel lines of L5 L4
  measures "d112" diameter of A0
  measures "d116" distance of L4.end L15.end
  measures "d117" distance of L14.end L15.end
  measures "d118" distance of L14.end L4.start
  measures "d119" distance between parallel lines of L0 L4
extrude "StuffplateMount" add sketch "stuffplate_Mount" against normal blind 6 contours L4 L1 L5 L3 | A0 | A1
sketch "Sketch8" plane through (90.804, 0, -64.1122) normal (0, 0, -1) x (-1, 0, 0)
  line L0 (179, 106) -> (4, 106)
  line L1 (4, 106) -> (4, 98)
  line L2 (4, 98) -> (179, 98)
  line L3 (179, 98) -> (179, 106)
  point P0 (90.804, 0)
  dimension "d122" = 8
  dimension "d123" = 175
  constraints: 8 end point, 2 parallel, 1 horizontal, 1 perpendicular
  measures "d122" distance between parallel lines of L2 L0
  measures "d123" distance between parallel lines of L3 L1
extrude "StuffplateMount2" add sketch "Sketch8" against normal blind 6
hole "Hole2" at (-92.196, 131, 48.8878) at (90.804, 0, 48.8878) at (-17.196, 102, 48.8878) at (42.804, 102, 48.8878) direction (0, 0, -1) diameter 2.1 end through all
body "Solid1"
